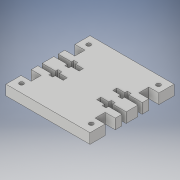
# Autodesk Inventor part: wall-front
Saved by Autodesk Inventor 2017 (Build 210142000, 142)
## iProperties
Created: 2017-02-28
Part Number: wall-front
Material: Generic
Document SubType Name: Modeling
Designer: John
Density: 1 g/cm^3
Appearance: Default
Author: John
Autodesk Inventor part; units mm, degrees
ref_plane "YZ Plane" through (0, 0, 0) normal (1, 0, 0) x (0, 1, 0)
ref_plane "XZ Plane" through (0, 0, 0) normal (0, 1, 0) x (-1, 0, 0)
ref_plane "XY Plane" through (0, 0, 0) normal (0, 0, 1) x (1, 0, 0)
sketch "Sketch1" plane through (0, 0, 0) normal (0, 1, 0) x (-1, 0, 0)
  line L0 (0, 0) -> (-50, 0)
  line L1 (-50, -50) -> (0, -50)
  line L2 (-50, -41) -> (-44, -41)
  line L3 (-44, -41) -> (-44, -35)
  line L4 (-44, -35) -> (-50, -35)
  line L5 (-50, -35) -> (-50, -41) construction
  line L6 (-50, -9) -> (-44, -9)
  line L7 (-44, -9) -> (-44, -15)
  line L8 (-44, -15) -> (-50, -15)
  line L9 (-50, -15) -> (-50, -9) construction
  line L10 (-25, 0) -> (-25, -50) construction
  line L11 (-50, -9) -> (-50, 0)
  line L12 (-50, -15) -> (-50, -19)
  line L13 (-50, -41) -> (-50, -50)
  circle A0 centre (-45.75, -5) radius 1.25
  circle A1 centre (-45.75, -45) radius 1.25
  line L14 (-50, -31) -> (-42, -31)
  line L15 (-35, -31) -> (-35, -28.5)
  line L16 (-35, -28.5) -> (-39.7, -28.5)
  line L17 (-50, -19) -> (-42, -19)
  line L18 (-35, -19) -> (-35, -21.5)
  line L19 (-35, -21.5) -> (-39.7, -21.5)
  line L20 (-50, -31) -> (-50, -35)
  line L21 (-50, -28.5) -> (-50, -31) construction
  line L22 (-50, -21.5) -> (-50, -28.5)
  line L23 (-50, -19) -> (-50, -21.5) construction
  line L24 (-42, -32.45) -> (-39.7, -32.45)
  line L25 (-39.7, -32.45) -> (-39.7, -31)
  line L26 (-39.7, -27.05) -> (-42, -27.05)
  line L27 (-42, -27.05) -> (-42, -28.5)
  line L28 (-42, -31) -> (-42, -32.45)
  line L29 (-42, -28.5) -> (-42, -31) construction
  line L30 (-42, -22.95) -> (-39.7, -22.95)
  line L31 (-39.7, -22.95) -> (-39.7, -21.5)
  line L32 (-39.7, -17.55) -> (-42, -17.55)
  line L33 (-42, -17.55) -> (-42, -19)
  line L34 (-42, -21.5) -> (-42, -22.95)
  line L35 (-42, -19) -> (-42, -21.5) construction
  line L36 (-39.7, -28.5) -> (-39.7, -27.05)
  line L37 (-39.7, -31) -> (-39.7, -28.5) construction
  line L38 (-39.7, -21.5) -> (-39.7, -19) construction
  line L39 (-39.7, -19) -> (-39.7, -17.55)
  line L40 (-42, -31) -> (-39.7, -31) construction
  line L41 (-39.7, -31) -> (-35, -31)
  line L42 (-42, -28.5) -> (-50, -28.5)
  line L43 (-39.7, -28.5) -> (-42, -28.5) construction
  line L44 (-42, -21.5) -> (-50, -21.5)
  line L45 (-39.7, -21.5) -> (-42, -21.5) construction
  line L46 (-42, -19) -> (-39.7, -19) construction
  line L47 (-39.7, -19) -> (-35, -19)
  line L48 (0, -41) -> (-6, -41)
  line L49 (-6, -41) -> (-6, -35)
  line L50 (-6, -35) -> (0, -35)
  line L51 (0, -35) -> (0, -41) construction
  line L52 (0, -9) -> (-6, -9)
  line L53 (-6, -9) -> (-6, -15)
  line L54 (-6, -15) -> (0, -15)
  line L55 (0, -15) -> (0, -9) construction
  line L56 (0, -9) -> (0, 0)
  line L57 (0, -15) -> (0, -19)
  line L58 (0, -41) -> (0, -50)
  circle A2 centre (-4.25, -5) radius 1.25
  circle A3 centre (-4.25, -45) radius 1.25
  line L59 (0, -31) -> (-8, -31)
  line L60 (-15, -31) -> (-15, -28.5)
  line L61 (-15, -28.5) -> (-10.3, -28.5)
  line L62 (0, -19) -> (-8, -19)
  line L63 (-15, -19) -> (-15, -21.5)
  line L64 (-15, -21.5) -> (-10.3, -21.5)
  line L65 (0, -31) -> (0, -35)
  line L66 (0, -28.5) -> (0, -31) construction
  line L67 (0, -21.5) -> (0, -28.5)
  line L68 (0, -19) -> (0, -21.5) construction
  line L69 (-8, -32.45) -> (-10.3, -32.45)
  line L70 (-10.3, -32.45) -> (-10.3, -31)
  line L71 (-10.3, -27.05) -> (-8, -27.05)
  line L72 (-8, -27.05) -> (-8, -28.5)
  line L73 (-8, -31) -> (-8, -32.45)
  line L74 (-8, -28.5) -> (-8, -31) construction
  line L75 (-8, -22.95) -> (-10.3, -22.95)
  line L76 (-10.3, -22.95) -> (-10.3, -21.5)
  line L77 (-10.3, -17.55) -> (-8, -17.55)
  line L78 (-8, -17.55) -> (-8, -19)
  line L79 (-8, -21.5) -> (-8, -22.95)
  line L80 (-8, -19) -> (-8, -21.5) construction
  line L81 (-10.3, -28.5) -> (-10.3, -27.05)
  line L82 (-10.3, -31) -> (-10.3, -28.5) construction
  line L83 (-10.3, -21.5) -> (-10.3, -19) construction
  line L84 (-10.3, -19) -> (-10.3, -17.55)
  line L85 (-8, -31) -> (-10.3, -31) construction
  line L86 (-10.3, -31) -> (-15, -31)
  line L87 (-8, -28.5) -> (0, -28.5)
  line L88 (-10.3, -28.5) -> (-8, -28.5) construction
  line L89 (-8, -21.5) -> (0, -21.5)
  line L90 (-10.3, -21.5) -> (-8, -21.5) construction
  line L91 (-8, -19) -> (-10.3, -19) construction
  line L92 (-10.3, -19) -> (-15, -19)
  dimension "d0" = 50
  dimension "d1" = 50
  dimension "d20" = 6
  dimension "d21" = 6
  dimension "d22" = 6
  dimension "d26" = 20
  dimension "d27" = 2.5
  dimension "d28" = 4.25
  dimension "d30" = 2.5
  dimension "d31" = 4.25
  dimension "d32" = 4
  dimension "d33" = 15
  dimension "d34" = 2.5
  dimension "d35" = 15
  dimension "d36" = 2.5
  dimension "d37" = 4
  dimension "d38" = 5.4
  dimension "d39" = 2.3
  dimension "d40" = 8
  dimension "d41" = 2.3
  dimension "d42" = 5.4
  dimension "d43" = 8
  dimension "d44" = 4
  constraints: 186 end point, 44 parallel, 34 symmetric about line, 14 collinear, 14 perpendicular, 11 horizontal, 6 point on line, 4 centre point, 2 midpoint, 1 vertical, 2 other
  measures "d0" distance of L1.end L1.start
  measures "d1" distance of L0.end L1.start
  measures "d20" distance of L4.end L3.end
  measures "d21" distance of L3.end L2.end
  measures "d22" distance of L6.end L7.end
  measures "d26" distance of L8.end L4.end
  measures "d27" diameter of A0
  measures "d28" distance from line of L11 A0.centre
  measures "d30" diameter of A1
  measures "d31" distance from line of L13 A1.centre
  measures "d32" distance from line of L2 A1.centre
  measures "d33" distance of L21.start L15.end
  measures "d34" distance of L15.end L15.start
  measures "d35" distance of L18.end L22.start
  measures "d36" distance of L18.start L18.end
  measures "d37" distance of L14.start L4.end
  measures "d38" distance of L24.end L26.start
  measures "d39" distance of L24.start L24.end
  measures "d40" distance between parallel lines of L21 L29
  measures "d41" distance of L32.end L32.start
  measures "d42" distance of L32.start L30.end
  measures "d43" distance between parallel lines of L23 L35
  measures "d44" distance from line of A0.centre L6
extrude "Extrusion2" add sketch "Sketch1" along normal blind 6
equation "\"d22\" = d21"
equation "\"d30\" = d27"
equation "\"d31\" = d28"
equation "\"d32\" = d44"
equation "\"d33\" = d35"
equation "\"d34\" = d27"
equation "\"d36\" = d27"
equation "\"d43\" = d40"
body "Solid2"
